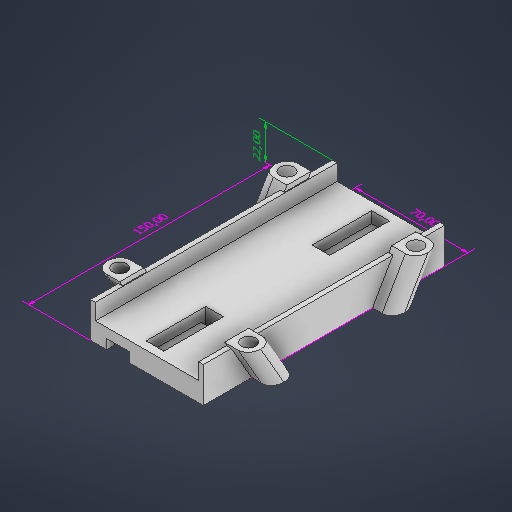
# Autodesk Inventor part: BaseCabina
Saved by Autodesk Inventor 2026.1 (Build 301233020, 233B)
## iProperties
Created: 2025-10-09
Part Number: BaseCabina
Material: Generic
Document SubType Name: Modeling
Designer: tito.luyo
Density: 1 g/cm^3
Appearance: Default
Author: tito.luyo
Autodesk Inventor part; units mm, degrees
ref_plane "YZ Plane" through (0, 0, 0) normal (1, 0, 0) x (0, 1, 0)
ref_plane "XZ Plane" through (0, 0, 0) normal (0, 1, 0) x (-1, 0, 0)
ref_plane "XY Plane" through (0, 0, 0) normal (0, 0, 1) x (1, 0, 0)
sketch "SketchBase" plane through (0, 0, 0) normal (0, 1, 0) x (-1, 0, 0)
  line L0 (0, 0) -> (70, 0)
  line L1 (70, 0) -> (70, -150)
  line L2 (70, -150) -> (0, -150)
  line L3 (0, -150) -> (0, 0)
  dimension "cabina_ancho" = 70
  dimension "cabina_largo" = 150
  constraints: 8 end point, 2 parallel, 1 horizontal, 1 perpendicular
  measures "cabina_ancho" distance of L1.end L2.end
  measures "cabina_largo" distance of L0.end L1.end
extrude "Base" add sketch "SketchBase" along normal blind 12
sketch "SketchBateria" plane through (0, 0, 0) normal (0, -1, 0) x (1, 0, 0)
  line L0 (-10, -60) -> (-31, -60)
  line L1 (-31, -60) -> (-31, -91)
  line L2 (-31, -91) -> (-10, -91)
  line L3 (-10, -91) -> (-10, -60)
  line L4 (0, 0) -> (0, -150) projected
  line L5 (-70, 0) -> (0, 0) projected
  point P0 (-20.5, -60)
  dimension "bateria_ancho" = 21
  dimension "bateria_largo" = 31
  dimension "bateria_sep_lateral" = 10
  dimension "bateria_sep_fondo" = 60
  constraints: 8 end point, 2 parallel, 1 horizontal, 1 midpoint, 1 perpendicular
  measures "bateria_ancho" distance of L2.end L1.end
  measures "bateria_largo" distance of L1.end L0.end
  measures "bateria_sep_lateral" distance between parallel lines of L4 L3
  measures "bateria_sep_fondo" distance from line of point (-20.5, -60) L5
extrude "Bateria" cut sketch "SketchBateria" against normal blind 7
sketch "SketchMicroControlador" plane through (0, 0, 0) normal (0, -1, 0) x (1, 0, 0)
  line L0 (-43, -5) -> (-63, -5)
  line L1 (-63, -5) -> (-63, -35)
  line L2 (-63, -35) -> (-43, -35)
  line L3 (-43, -35) -> (-43, -5)
  line L4 (-70, -150) -> (-70, 0) projected
  line L5 (-70, 0) -> (0, 0) projected
  dimension "micro_ancho" = 20
  dimension "micro_largo" = 30
  dimension "micro_sep_lateral" = 7
  dimension "micro_sep_fondo" = 5
  constraints: 8 end point, 2 parallel, 1 horizontal, 1 perpendicular
  measures "micro_ancho" distance of L2.end L1.end
  measures "micro_largo" distance of L1.end L0.end
  measures "micro_sep_lateral" distance between parallel lines of L4 L1
  measures "micro_sep_fondo" distance between parallel lines of L5 L0
extrude "MicroControlador" cut sketch "SketchMicroControlador" against normal blind 6
sketch "SketchSensorPresencia" plane through (0, 12, 0) normal (0, 1, 0) x (1, 0, 0)
  line L0 (-29.5, 108) -> (-40.5, 108)
  line L1 (-40.5, 108) -> (-40.5, 145)
  line L2 (-40.5, 145) -> (-29.5, 145)
  line L3 (-29.5, 145) -> (-29.5, 108)
  line L4 (0, 150) -> (-70, 150) projected
  line L5 (0, 0) -> (0, 150) projected
  point P0 (-35, 150)
  point P1 (-35, 145)
  dimension "presencia_ancho" = 11
  dimension "presencia_largo" = 37
  dimension "presencia_sep_fondo" = 5
  dimension "presencia_sep_lateral" = 29.5
  constraints: 8 end point, 2 midpoint, 2 parallel, 1 horizontal, 1 perpendicular
  measures "presencia_ancho" distance of L1.end L2.end
  measures "presencia_largo" distance of L0.end L1.end
  measures "presencia_sep_fondo" distance of point (-35, 150) point (-35, 145)
  measures "presencia_sep_lateral" distance between parallel lines of L5 L3
extrude "SensorPresencia" cut sketch "SketchSensorPresencia" against normal blind 7
sketch "SketchSoporte" plane through (0, 0, 0) normal (0, -1, 0) x (1, 0, 0)
  line L0 (12.5, -45) -> (-2.5, -45)
  line L1 (-2.5, -45) -> (-2.5, -30)
  line L2 (-2.5, -30) -> (12.5, -30)
  line L3 (12.5, -30) -> (12.5, -45)
  line L4 (-70, 0) -> (0, 0) projected
  line L5 (0, 0) -> (0, -150) projected
  dimension "soporte_ancho" = 15
  dimension "soporte_largo" = 15
  dimension "soporte_sep_extremo" = 30
  dimension "soporte_ins_lateral" = 12.5
  constraints: 8 end point, 2 parallel, 1 horizontal, 1 perpendicular
  measures "soporte_ancho" distance of L1.end L2.end
  measures "soporte_largo" distance of L0.end L1.end
  measures "soporte_sep_extremo" distance between parallel lines of L2 L4
  measures "soporte_ins_lateral" distance between parallel lines of L5 L3
sketch "SketchSoporteGuiaInclinada" plane through (0, 0, 0) normal (1, 0, 0) x (0, 0, -1)
  line L0 (150, 0) -> (0, 0) projected
  line L1 (20, 0) -> (5.5662, 25)
  dimension "soporte_guia_sep_extremo" = 20
  dimension "soporte_guia_inclinacion" = 60
  dimension "soporte_guia_altura" = 25
  constraints: 2 end point, 1 point on line
  measures "soporte_guia_sep_extremo" distance of L0.end L1.start
  measures "soporte_guia_inclinacion" angle of L0 L1
  measures "soporte_guia_altura" distance from line of L0 L1.end
sweep "Soporte" add profiles "SketchSoporte" path "SketchSoporteGuiaInclinada" path curves L1
sketch "SketchSoporteHueco" plane through (-2.5, 25, -15.5662) normal (0, 1, 0) x (1, 0, 0)
  circle A0 centre (7.5, 7.5) radius 4.45
  line L0 (15, 15) -> (0, 15) projected
  line L1 (0, 15) -> (0, 0) projected
  point P0 (2.5, -15.5662)
  dimension "soporte_hueco_diametro" = 8.9
  dimension "soporte_hueco_sep_largo" = 7.5
  dimension "soporte_hueco_sep_ancho" = 7.5
  constraints: 1 centre point
  measures "soporte_hueco_diametro" diameter of A0
  measures "soporte_hueco_sep_largo" distance from line of L0 A0.centre
  measures "soporte_hueco_sep_ancho" distance from line of L1 A0.centre
sketch3d "3D Sketch_guia_soporteHueco"
  line L0 (12.5, 25, -30.5662) -> (12.5, 0, -45)
sweep "SoporteHueco" cut profiles "SketchSoporteHueco" path "3D Sketch_guia_soporteHueco"
sketch "SketchGuiasMitadPlano" plane through (0, 0, 0) normal (0, -1, 0) x (1, 0, 0)
  line L0 (-35, -155.1159) -> (-35, 14.8841) construction
  line L1 (-70, -150) -> (-70, 0) construction
  line L2 (14.1346, -75) -> (-95.8654, -75) construction
  line L3 (0, -150) -> (-70, -150) construction
  point P0 (0, 0)
  dimension "guia_mitad_ancho_longitud" = 170
  dimension "guia_mitad_ancho_posicion" = 35
  dimension "guia_mitad_largo_longitud" = 110
  dimension "guia_mitad_largo_posicion" = 75
  constraints: 4 end point, 1 horizontal, 1 vertical
  measures "guia_mitad_ancho_longitud" distance of L0.start L0.end
  measures "guia_mitad_ancho_posicion" distance between parallel lines of L1 L0
  measures "guia_mitad_largo_longitud" distance of L2.start L2.end
  measures "guia_mitad_largo_posicion" distance between parallel lines of L3 L2
ref_plane "Work Plane Vertical Medio" through (0, 0, -75) normal (0, 0, -1) x (-1, 0, 0)
sketch "SketchGuiaVerticalCentral" plane through (0, 0, -75) normal (0, 0, -1) x (-1, 0, 0)
  line L0 (35, 32.2596) -> (35, -17.7404)
  line L1 (70, 0) -> (70, 12) construction
  point P0 (0, 0)
  dimension "guia_centro_vertical_longitud" = 50
  dimension "guia_centro_vertical_posicion" = 35
  constraints: 2 end point, 1 vertical
  measures "guia_centro_vertical_longitud" distance of L0.start L0.end
  measures "guia_centro_vertical_posicion" distance between parallel lines of L1 L0
ref_plane "Work Plane Horiz Medio" through (-35, 0, -150) normal (-1, 0, 0) x (0, 0, 1)
mirror "SensorPresencia2" about plane through (0, 0, -75) normal (0, 0, -1) of "SensorPresencia"
sketch "SketchUsbSock" plane through (0, 0, 0) normal (0, -1, 0) x (1, 0, 0)
  line L0 (-46, -5) -> (-60, -5)
  line L1 (-60, -5) -> (-60, 0)
  line L2 (-60, 0) -> (-46, 0)
  line L3 (-46, 0) -> (-46, -5)
  line L4 (-70, -150) -> (-70, 0) projected
  line L5 (-63, -5) -> (-43, -5) projected
  point P0 (0, 0)
  point P1 (-80, -30)
  dimension "micro_usbsock_largo" = 5
  dimension "micro_usbsock_ancho" = 14
  dimension "micro_usbsock_sep_lateral" = 10
  constraints: 8 end point, 2 parallel, 1 collinear, 1 horizontal, 1 perpendicular, 1 other
  measures "micro_usbsock_largo" distance between parallel lines of L2 L0
  measures "micro_usbsock_ancho" distance between parallel lines of L1 L3
extrude "Extrusion7" cut sketch "SketchUsbSock" against normal blind 6
fillet "SoporteRedondeado1" radius 6.5 1 edges at (12.5, 12.5, -22.7831)
fillet "SoporteRedondeado2" radius 6.5 1 edges at (12.5, 12.5, -37.7831)
mirror "Mirror4" about plane through (-35, 0, -150) normal (-1, 0, 0) of "Soporte", "SoporteHueco", "SoporteRedondeado1", "SoporteRedondeado2"
mirror "Mirror5" about plane through (0, 0, -75) normal (0, 0, -1) of "SoporteHueco", "Soporte", "SoporteRedondeado2", "SoporteRedondeado1", "Mirror4"
sketch "Sketch15" plane through (0, 0, 0) normal (0, -1, 0) x (1, 0, 0)
  line L0 (-50, -117.5) -> (-65, -117.5)
  line L1 (-65, -117.5) -> (-65, -145)
  line L2 (-65, -145) -> (-50, -145)
  line L3 (-50, -145) -> (-50, -117.5)
  line L4 (0, -150) -> (-70, -150) projected
  line L5 (-70, -150) -> (-70, -120) projected
  point P0 (0, 0)
  dimension "sensordistancia_ancho" = 15
  dimension "sensordistancia_largo" = 27.5
  dimension "sensordistancia_sep_fondo" = 5
  dimension "sensordistancia_sep_lateral" = 5
  constraints: 8 end point, 2 parallel, 1 horizontal, 1 perpendicular
  measures "sensordistancia_ancho" distance of L2.end L1.end
  measures "sensordistancia_largo" distance of L1.end L0.end
  measures "sensordistancia_sep_fondo" distance between parallel lines of L4 L2
  measures "sensordistancia_sep_lateral" distance between parallel lines of L5 L1
extrude "SensorDistancia" cut sketch "Sketch15" against normal blind 5
sketch "Sketch16" plane through (0, 12, 0) normal (0, 1, 0) x (1, 0, 0)
  line L0 (-3, 0) -> (0, 0)
  line L1 (0, 0) -> (0, 150)
  line L2 (0, 150) -> (-3, 150)
  line L3 (-3, 150) -> (-3, 0)
  line L4 (0, 150) -> (-70, 150) projected
  line L5 (0, 126.9282) -> (0, 150) projected
  line L6 (-70, 0) -> (0, 0) projected
  line L7 (-70, 0) -> (-67, 0)
  line L8 (-67, 0) -> (-67, 150)
  line L9 (-67, 150) -> (-70, 150)
  line L10 (-70, 150) -> (-70, 0)
  line L11 (-70, 23.0718) -> (-70, 0) projected
  dimension "pared_lateral_1_ancho" = 3
  dimension "pared_lateral_2_ancho" = 3
  constraints: 16 end point, 6 collinear, 4 parallel, 2 horizontal, 2 perpendicular
  measures "pared_lateral_1_ancho" distance of L2.end L1.end
  measures "pared_lateral_2_ancho" distance of L9.end L8.end
extrude "ParedesLaterales" add sketch "Sketch16" along normal blind 10 contours L3 L2 L1 L0 | L6 L10 L4 L8
sketch "Sketch17" plane through (0, 5, 0) normal (0, 1, 0) x (1, 0, 0)
  line L0 (-29.5, 108) -> (-40.5, 108)
  line L1 (-40.5, 108) -> (-40.5, 111)
  line L2 (-40.5, 111) -> (-29.5, 111)
  line L3 (-29.5, 111) -> (-29.5, 108)
  line L4 (-29.5, 108) -> (-40.5, 108) projected
  line L5 (-29.5, 145) -> (-29.5, 108) projected
  line L6 (-40.5, 108) -> (-40.5, 145) projected
  point P0 (0, 0)
  dimension "presencia_cables_hueco_ancho" = 3
  constraints: 8 end point, 3 collinear, 2 parallel, 1 horizontal, 1 perpendicular
  measures "presencia_cables_hueco_ancho" distance of L0.end L1.end
extrude "presencia_hueco" cut sketch "Sketch17" against normal blind 5
mirror "Mirror6" about plane through (0, 0, -75) normal (0, 0, -1) of "presencia_hueco"
equation "\"presencia_sep_lateral\" = -0.5 * presencia_ancho + 0.5 * cabina_ancho"
equation "\"soporte_hueco_sep_largo\" = 0.5 * soporte_largo"
equation "\"soporte_hueco_sep_ancho\" = 0.5 * soporte_ancho"
equation "\"guia_mitad_ancho_posicion\" = 0.5 * cabina_ancho"
equation "\"guia_mitad_largo_posicion\" = 0.5 * cabina_largo"
equation "\"guia_centro_vertical_posicion\" = 0.5 * cabina_ancho"
equation "\"micro_usbsock_largo\" = micro_sep_fondo"
equation "\"micro_usbsock_sep_lateral\" = micro_sep_lateral + 0.5 * micro_ancho - 0.5 * micro_usbsock_ancho"
equation "\"micro_usbsock_espesor\" = micro_espesor"
equation "\"soporte_redondeado2\" = soporte_redondeado1"
equation "\"presencia_cables_hueco_espesor\" = cabina_espesor - presencia_espesor"
equation "\"llantas_distancia_ejes\" = 89"
equation "\"llantas_distancia_ancho\" = 47"
equation "\"llantas_ancho\" = 8.5"
equation "\"llantas_diametro\" = 25.6"
equation "\"soporte_hueco_tolerancia\" = 0.9"
equation "\"micro_espesor\" = 6"
equation "\"soporte_redondeado1\" = 6.5"
equation "\"cabina_espesor\" = 12"
equation "\"presencia_espesor\" = 7"
body "Solid1"
